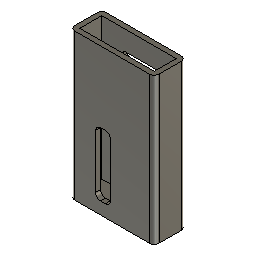
Hayabusa Quickshifter Housing (Autodesk Fusion 360 design; units mm, degrees)
Autodesk Fusion 360 part; units mm, degrees
note: some values were not read from the file. Set by a fixed rule: which sketch regions a step uses.
sketch "Skizze1" plane through (0, 0, 0) normal (0, 0, 1) x (1, 0, 0)
  line L0 (15.25, -4.5) -> (-15.25, -4.5)
  line L1 (-15.25, -4.5) -> (-15.25, 4.5)
  line L2 (-15.25, 4.5) -> (15.25, 4.5)
  line L3 (15.25, 4.5) -> (15.25, -4.5)
  line L4 (15.25, -4.5) -> (-15.25, 4.5) construction
  line L5 (-15.25, -4.5) -> (15.25, 4.5) construction
  line L6 (17.25, -6.5) -> (-17.25, -6.5)
  line L7 (-17.25, -6.5) -> (-17.25, 6.5)
  line L8 (-17.25, 6.5) -> (17.25, 6.5)
  line L9 (17.25, 6.5) -> (17.25, -6.5)
  line L10 (17.25, -6.5) -> (-17.25, 6.5) construction
  line L11 (-17.25, -6.5) -> (17.25, 6.5) construction
  dimension "d1" = 30.5
  dimension "d2" = 9
  dimension "d3" = 34.5
  dimension "d4" = 13
  constraint horizontal L0
  constraint perpendicular L0 L1
  constraint parallel L0 L2
  constraint parallel L1 L3
  constraint coincident L4 origin
  constraint coincident L5 origin
  constraint horizontal L6
  constraint perpendicular L6 L7
  constraint parallel L6 L8
  constraint parallel L7 L9
  constraint coincident L10 origin
  constraint coincident L11 origin
  measures "d1" distance of L1.end L2.end
  measures "d2" distance of L0.end L1.end
  measures "d3" distance of L7.end L8.end
  measures "d4" distance of L6.end L7.end
extrude "Extrusion1" add sketch "Skizze1" against normal blind 2 contours L0 L1 L2 L3 | L6 L7 L8 L9
extrude "Extrusion2" add sketch "Skizze1" along normal blind 58
fillet "Abrundung1" radius 2 4 edges at (-17.25, -6.5, 28) (-17.25, 6.5, 28) (17.25, -6.5, 28) (17.25, 6.5, 28)
sketch "Skizze2" plane through (0, -6.5, 0) normal (0, -1, 0) x (1, 0, 0)
  line L0 (15.25, -2) -> (15.25, 58)
  line L1 (15.25, 58) -> (-15.25, 58)
  line L2 (-15.25, 58) -> (-15.25, -2)
  line L3 (-15.25, -2) -> (15.25, -2)
  line L4 (-6.75, 3) -> (-0.75, 3)
  line L5 (-0.75, 3) -> (-0.75, 29)
  line L6 (-0.75, 29) -> (-6.75, 29)
  line L7 (-6.75, 29) -> (-6.75, 3)
  line L8 (-17.25, 58) -> (-17.25, -2)
  line L9 (17.25, 0) -> (-17.25, 0)
  dimension "d11" = 6
  dimension "d12" = 26
  dimension "d19" = 8.5
  dimension "d20" = 3
  constraint horizontal L4
  constraint vertical L5
  constraint horizontal L6
  constraint vertical L7
  measures "d11" distance of L4.start L4.end
  measures "d12" distance of L4.start L6.end
  measures "d19" distance of L2 L7
  measures "d20" distance of L4 L9
extrude "Extrusion3" cut sketch "Skizze2" against normal blind 2 contours L4 L5 L6 L7
fillet "Abrundung2" radius 2 4 edges at (-0.75, -5.5, 29) (-6.75, -5.5, 29) (-0.75, -5.5, 3) (-6.75, -5.5, 3)
sketch "Skizze3" plane through (0, 6.5, 0) normal (0, 1, 0) x (-1, 0, 0)
  line L0 (-15.25, 58) -> (-15.25, -2)
  line L1 (-15.25, -2) -> (15.25, -2)
  line L2 (15.25, -2) -> (15.25, 58)
  line L3 (15.25, 58) -> (-15.25, 58)
  line L4 (-12.25, 50) -> (5.75, 50)
  line L5 (6.75, 49) -> (6.75, 48)
  line L6 (5.75, 47) -> (-12.25, 47)
  line L7 (-13.25, 48) -> (-13.25, 49)
  line L8 (-15.25, 0) -> (15.25, 0)
  arc A0 (-12.25, 50) -> (-13.25, 49) centre (-12.25, 49) ccw
  arc A1 (-13.25, 48) -> (-12.25, 47) centre (-12.25, 48) ccw
  arc A2 (5.75, 47) -> (6.75, 48) centre (5.75, 48) ccw
  arc A3 (6.75, 49) -> (5.75, 50) centre (5.75, 49) ccw
  point P0 (-13.25, 50)
  point P1 (6.75, 50)
  dimension "d21" = 47
  dimension "d22" = 50
  dimension "d23" = 20
  dimension "d24" = 2
  dimension "d27" = 1
  constraint horizontal L4
  constraint vertical L5
  constraint horizontal L6
  constraint vertical L7
  constraint coincident P0 L4
  constraint coincident P0 L7
  constraint tangent L4 A0
  constraint tangent L7 A0
  constraint tangent L6 A1
  constraint tangent L7 A1
  constraint equal A0 A1
  constraint tangent L5 A2
  constraint tangent L6 A2
  constraint equal A0 A2
  constraint coincident P1 L4
  constraint coincident P1 L5
  constraint tangent L4 A3
  constraint tangent L5 A3
  constraint equal A0 A3
  measures "d21" distance of L6 L8
  measures "d22" distance of L4 L8
  measures "d23" distance of P0 P1
  measures "d24" distance of L0 L7
  measures "d27" radius of A0
extrude "Extrusion4" cut sketch "Skizze3" against normal blind 3 contours L4 L5 L6 L7 A0 A1 A2 A3
equation "d3 = d1 + ( ( 2 * 2 ) * 1 mm )"
equation "d4 = d2 + ( ( 2 * 2 ) * 1 mm )"
equation "d12 = 28 mm - 2 mm"
